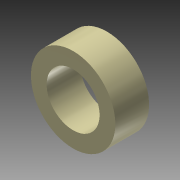
# Autodesk Inventor part: Nylon Spacer 1_8th
Saved by Autodesk Inventor 2014 SP1 (Build 180222100, 222)
## iProperties
Created: 2016-04-12
Part Number: Nylon Spacer 1_8th
Material: Generic
Document SubType Name: Modeling
Designer: Ben
Density: 1 g/cm^3
Appearance: Default
Author: Ben
Autodesk Inventor part; units mm, degrees
ref_plane "YZ Plane" through (0, 0, 0) normal (1, 0, 0) x (0, 1, 0)
ref_plane "XZ Plane" through (0, 0, 0) normal (0, 1, 0) x (-1, 0, 0)
ref_plane "XY Plane" through (0, 0, 0) normal (0, 0, 1) x (1, 0, 0)
sketch "Sketch1" plane through (0, 0, 0) normal (1, 0, 0) x (0, 1, 0)
  line L0 (2.4892, 3.175) -> (3.9687, 3.175)
  line L1 (3.9687, 3.175) -> (3.9687, 0)
  line L2 (3.9687, 0) -> (2.4892, 0)
  line L3 (2.4892, 0) -> (2.4892, 3.175)
  line L4 (0, 0) -> (0, 12.9411) construction
  dimension "d0" = 3.175
  dimension "d1" = 4.9784
  dimension "d2" = 7.9375
  constraints: 10 end point, 3 parallel, 1 horizontal, 1 perpendicular, 1 point on line
  measures "d0" distance of L0.end L1.end
  measures "d1" diameter of L3 L4
  measures "d2" diameter of L1 L4
revolve "Revolution1" add sketch "Sketch1" angle 360 about axis through (0, 0, 0) along (0, 0, 1)
body "Solid1"
